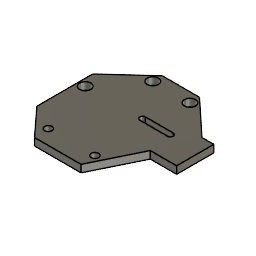
Diagram-2(11) (Autodesk Fusion 360 design; units mm, degrees)
part number: 2026-03-10-21-09-01-468
Autodesk Fusion 360 part; units mm, degrees
sketch "Sketch1" plane through (0, 0, 0) normal (0, 0, 1) x (1, 0, 0)
  line L0 (-4.1621, 53.0041) -> (15.8379, 53.0041)
  line L1 (15.2055, -10.0393) -> (-9.7945, -10.0393)
  line L2 (-23.7204, 35.1678) -> (-23.7204, 5.1678)
  line L3 (-9.7945, -10.0393) -> (-23.7204, 5.1678)
  line L4 (-23.7204, 35.1678) -> (-4.1621, 53.0041)
  line L5 (27.3696, 14.9582) -> (41.5696, 14.9582)
  line L6 (15.2055, -10.0393) -> (27.3696, 14.9582)
  line L7 (41.5696, 14.9582) -> (41.5696, 34.9582)
  line L8 (41.5696, 34.9582) -> (35.203, 34.9582)
  line L9 (15.8379, 53.0041) -> (35.203, 34.9582)
  circle A0 centre (-19.9893, 27.4235) radius 3
  circle A1 centre (-10.1705, -2.1928) radius 2
  circle A2 centre (14.8295, -2.1928) radius 2
  line L10 (10.4224, 29.2929) -> (25.4224, 29.2929)
  line L11 (10.4224, 26.2929) -> (25.4224, 26.2929)
  arc A3 (10.4224, 29.2929) -> (10.4224, 26.2929) centre (10.4224, 27.7929) ccw
  arc A4 (25.4224, 26.2929) -> (25.4224, 29.2929) centre (25.4224, 27.7929) ccw
  circle A5 centre (-4.1621, 47.8544) radius 3
  circle A6 centre (15.8379, 47.8544) radius 3
  dimension "d1" = 20
  dimension "d3" = 25
  dimension "d4" = 30
  dimension "d5" = 20.62
  dimension "d6" = 26.47
  dimension "d7" = 14.2
  dimension "d8" = 27.8
  dimension "d9" = 20
  dimension "d10" = 26.47
  dimension "d13" = 6
  dimension "d14" = 4
  dimension "d15" = 4
  dimension "d16" = 3
  dimension "d17" = 3
  dimension "d18" = 15
  dimension "d19" = 65.29
  dimension "d20" = 6
  dimension "d21" = 6
  constraint horizontal L0
  constraint perpendicular L1 L2
  constraint perpendicular L5 L7
  constraint perpendicular L7 L8
  constraint coincident L9 L8.end
  constraint tangent L10 A4
  constraint tangent L11 A4
  constraint parallel L10 L11
  measures "d1" distance of L0.start L0.end
  measures "d3" distance of L1.start L1.end
  measures "d4" distance of L2.start L2.end
  measures "d5" distance of L1.end L2.end
  measures "d6" distance of L0.start L2.start
  measures "d7" distance of L5.start L5.end
  measures "d8" distance of L1.start L5.start
  measures "d9" distance of L5.end L7.end
  measures "d10" distance of L0.end L8.end
  measures "d13" diameter of A0
  measures "d14" diameter of A1
  measures "d15" diameter of A2
  measures "d16" diameter of A4
  measures "d17" diameter of A3
  measures "d18" distance of L10.start L10.end
  measures "d19" horizontal distance of L2.end L5.end
  measures "d20" diameter of A5
  measures "d21" diameter of A6
extrude "Extrude1" add sketch "Sketch1" along normal blind 4
